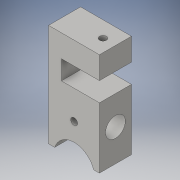
# Autodesk Inventor part: Over Support For Arm With Delrin
Saved by Autodesk Inventor 2016 (Build 200138000, 138)
## iProperties
Created: 2015-08-15
Part Number: Over Support For Arm With Delrin
Material: Generic
Document SubType Name: Modeling
Designer: steele
Density: 1 g/cm^3
Appearance: Default
Author: steele
Autodesk Inventor part; units mm, degrees
note: some values were not read from the file. Chosen so that the rebuilt part matches the saved one: direction of "Hole1".
ref_plane "YZ Plane" through (0, 0, 0) normal (1, 0, 0) x (0, 1, 0)
ref_plane "XZ Plane" through (0, 0, 0) normal (0, 1, 0) x (-1, 0, 0)
ref_plane "XY Plane" through (0, 0, 0) normal (0, 0, 1) x (1, 0, 0)
sketch "Sketch1" plane through (0, 0, 0) normal (0, 0, 1) x (1, 0, 0)
  line L0 (0, 0) -> (-50.8, 0)
  line L1 (-50.8, 0) -> (-50.8, -101.6)
  line L2 (-50.8, -101.6) -> (0, -101.6)
  line L3 (0, -22.225) -> (-38.1, -22.225)
  line L4 (-38.1, -22.225) -> (-38.1, -41.275)
  line L5 (-38.1, -41.275) -> (0, -41.275)
  line L6 (0, -101.6) -> (0, -41.275)
  line L7 (0, -22.225) -> (0, 0)
  dimension "d0" = 101.6
  dimension "d1" = 50.8
  dimension "d4" = 22.225
  dimension "d5" = 38.1
  dimension "d6" = 19.05
  constraints: 16 end point, 3 parallel, 2 horizontal, 2 perpendicular
  measures "d0" distance of L0.end L1.end
  measures "d1" distance of L0.start L0.end
  measures "d4" distance between parallel lines of L3 L0
  measures "d5" distance of L3.start L3.end
  measures "d6" distance between parallel lines of L5 L3
extrude "Extrusion1" add sketch "Sketch1" along normal blind 31.75
sketch "Sketch2" plane through (0, -22.225, 0) normal (1, 0, 0) x (0, 0, -1)
  line L0 (-31.75, 0) -> (-31.75, 22.225) projected
  line L1 (0, 22.225) -> (0, -79.375) projected
  line L2 (-31.75, 22.225) -> (0, 22.225)
  line L3 (0, 22.225) -> (0, -79.375)
  line L4 (0, -79.375) -> (-31.75, -79.375)
  line L5 (-31.75, -79.375) -> (-31.75, 22.225)
  constraints: 8 end point, 2 parallel, 1 horizontal, 1 perpendicular
extrude "Extrusion2" cut sketch "Sketch2" against normal blind 0.381
sketch "Sketch3" plane through (-50.8, 0, 31.75) normal (0, 1, 0) x (1, 0, 0)
  line L0 (0, 31.75) -> (0, 0) projected
  line L1 (50.419, 31.75) -> (0, 31.75) projected
  point P0 (50.8, 31.75)
  point P1 (38.1, 15.875)
  dimension "d9" = 38.1
  dimension "d10" = 15.875
  measures "d9" distance from line of L0 point (38.1, 15.875)
  measures "d10" distance from line of L1 point (38.1, 15.875)
hole "Hole1" at (-12.7, 0, 15.875) direction (0, -1, 0) diameter 6.7564 end up to surface clearance for "Flat Head Machine Screw (82)" size "1/4" standard "Ansi Unified Screw Threads"
sketch "Sketch4" plane through (-50.8, -101.6, 0) normal (-1, 0, 0) x (0, 0, 1)
  line L0 (0, 101.6) -> (0, 0) projected
  line L1 (0, 101.6) -> (31.75, 101.6) projected
  point P0 (15.875, 69.85)
  dimension "d18" = 15.875
  dimension "d19" = 31.75
  measures "d18" distance from line of L0 point (15.875, 69.85)
  measures "d19" distance from line of L1 point (15.875, 69.85)
hole "Hole2" at (-50.8, -31.75, 15.875) direction (1, 0, 0) diameter 6.7564 end through all clearance for "Hex Head Bolt" size "1/4" standard "Ansi Unified Screw Threads"
sketch "Sketch5" plane through (-50.8, -101.6, 0) normal (-1, 0, 0) x (0, 0, 1)
  line L0 (0, 101.6) -> (0, 0) projected
  line L1 (0, 101.6) -> (31.75, 101.6) projected
  point P0 (15.875, 31.75)
  dimension "d27" = 15.875
  dimension "d28" = 69.85
  measures "d27" distance from line of L0 point (15.875, 31.75)
  measures "d28" distance from line of L1 point (15.875, 31.75)
hole "Hole3" at (-50.8, -69.85, 15.875) direction (1, 0, 0) diameter 19.558 end through all
sketch "Sketch6" plane through (0, 0, 31.75) normal (0, 0, 1) x (1, 0, 0)
  line L0 (-0.381, 0) -> (-50.8, 0) projected
  line L1 (-50.8, 0) -> (-50.8, -101.6) projected
  point P0 (0, 0)
  point P1 (-25.4, -69.85)
  dimension "d36" = 69.85
  dimension "d37" = 25.4
  measures "d36" distance from line of L0 point (-25.4, -69.85)
  measures "d37" distance from line of L1 point (-25.4, -69.85)
hole "Hole4" at (-25.4, -69.85, 31.75) direction (0, 0, -1) diameter 6.7564 end through all clearance for "Hex Head Bolt" size "1/4" standard "Ansi Unified Screw Threads"
sketch "Sketch7" plane through (0, 0, 31.75) normal (0, 0, 1) x (1, 0, 0)
  circle A0 centre (-25.4, -107.95) radius 20.32
  line L0 (-0.381, 0) -> (-50.8, 0) projected
  line L1 (-50.8, 0) -> (-50.8, -101.6) projected
  point P0 (0, 0)
  dimension "d45" = 107.95
  dimension "d46" = 25.4
  dimension "d47" = 40.64
  constraints: 1 centre point
  measures "d45" distance from line of A0.centre L0
  measures "d46" distance from line of A0.centre L1
  measures "d47" diameter of A0
extrude "Extrusion3" cut sketch "Sketch7" against normal through all
equation "\"d10\" = 0.5 * width"
equation "\"d18\" = 0.5 * width"
equation "\"width\" = 31.75"
body "Solid1"
